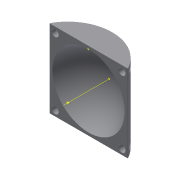
# Autodesk Inventor part: Custom Mirror Design
Saved by Autodesk Inventor 2015 (Build 190159000, 159)
## iProperties
Created: 2014-09-05
Part Number: Custom Mirror Design
Material: Generic
Document SubType Name: Modeling
Designer: I Rabey
Density: 1 g/cm^3
Appearance: Default
Author: I Rabey
Autodesk Inventor part; units mm, degrees
ref_plane "YZ Plane" through (0, 0, 0) normal (1, 0, 0) x (0, 1, 0)
sketch "Sketch11" plane through (0, 0, 0) normal (0, 0, 1) x (1, 0, 0)
  line L0 (-65, -65) -> (65, -65)
  line L1 (65, -65) -> (65, 65)
  line L2 (65, 65) -> (-65, 65)
  line L3 (-65, 65) -> (-65, -65)
  line L4 (-65, -65) -> (65, 65) construction
  line L5 (65, -65) -> (-65, 65) construction
  point P0 (0, 0)
  dimension "d36" = 130
  dimension "d37" = 130
  constraints: 12 end point, 2 midpoint, 2 parallel, 1 horizontal, 1 perpendicular
  measures "d36" distance of L2.end L1.end
  measures "d37" distance of L1.end L0.end
extrude "Extrusion5" add sketch "Sketch11" against normal blind 150
sketch "Sketch12" plane through (0, 0, 0) normal (0, 0, 1) x (1, 0, 0)
  arc A0 (0, 75) -> (0, -75) centre (0, 0) ccw
  line L0 (0, 0) -> (0, 75) construction
  line L1 (0, 0) -> (75, 0) construction
  line L2 (0, 0) -> (0, -75) construction
  line L3 (0, 75) -> (0, -75)
  dimension "d40" = 75
  dimension "d41" = 90
  dimension "d42" = 180
  constraints: 8 end point, 2 point on circle, 1 centre point, 1 coincident, 1 horizontal, 1 perpendicular
  measures "d40" radius of A0
  measures "d41" angle of L1 L0
  measures "d42" angle of L2 L0
revolve "Revolution5" cut sketch "Sketch12" angle 180 about axis through (0, 0, 0) along (0, -1, 0)
ref_plane "Work Plane2" through (0, 65, -37.4166) normal (0, 0, 1) x (1, 0, 0)
sketch "Sketch13" plane through (0, 65, -37.4166) normal (0, 0, 1) x (1, 0, 0)
  line L0 (-65, -130) -> (65, -130)
  line L1 (65, -130) -> (65, 0)
  line L2 (65, 0) -> (-65, 0)
  line L3 (-65, 0) -> (-65, -130)
  line L4 (-65, -130) -> (65, 0) construction
  line L5 (65, -130) -> (-65, 0) construction
  point P0 (0, -65)
  dimension "d45" = 130
  dimension "d46" = 130
  constraints: 12 end point, 2 midpoint, 2 parallel, 1 horizontal, 1 perpendicular
  measures "d45" distance of L2.end L1.end
  measures "d46" distance of L1.end L0.end
extrude "Extrusion6" cut sketch "Sketch13" along normal blind 50
sketch "Sketch14" plane through (0, 65, -37.4166) normal (0, 0, 1) x (1, 0, 0)
  line L0 (-65, -130) -> (65, -130)
  line L1 (65, -130) -> (65, 0)
  line L2 (65, 0) -> (-65, 0)
  line L3 (-65, 0) -> (-65, -130)
  line L4 (-65, -130) -> (65, 0) construction
  line L5 (65, -130) -> (-65, 0) construction
  line L6 (-70, -135) -> (70, -135)
  line L7 (70, -135) -> (70, 5)
  line L8 (70, 5) -> (-70, 5)
  line L9 (-70, 5) -> (-70, -135)
  line L10 (-70, -135) -> (70, 5) construction
  line L11 (70, -135) -> (-70, 5) construction
  point P0 (0, -65)
  dimension "d49" = 130
  dimension "d50" = 130
  dimension "d51" = 140
  dimension "d52" = 140
  constraints: 24 end point, 4 midpoint, 4 parallel, 2 horizontal, 2 perpendicular
  measures "d49" distance of L2.end L1.end
  measures "d50" distance of L1.end L0.end
  measures "d51" distance of L8.end L7.end
  measures "d52" distance of L7.end L6.end
extrude "Extrusion7" add sketch "Sketch14" against normal blind 75
sketch "Sketch17" plane through (0, 0, 0) normal (1, 0, 0) x (0, 1, 0)
  arc A0 (-80, 0) -> (80, 0) centre (0, 0) ccw
  line L0 (0, 0) -> (80, 0) construction
  line L1 (0, 0) -> (80, 0) construction
  line L2 (0, 0) -> (-80, 0) construction
  dimension "d57" = 80
  dimension "d58" = 0
  dimension "d59" = 180
  constraints: 6 end point, 2 point on circle, 1 centre point, 1 coincident, 1 collinear, 1 horizontal
  measures "d57" radius of A0
  measures "d58" distance between parallel lines of L0 L1
  measures "d59" angle of L2 L0
sketch "Sketch18" plane through (-65, 65, -150) normal (0, 1, 0) x (1, 0, 0)
  line L0 (0, -37.5834) -> (130, -37.5834)
  line L1 (130, -37.5834) -> (130, 0)
  line L2 (130, 0) -> (0, 0)
  line L3 (0, 0) -> (0, -37.5834)
  point P0 (65, -150)
  constraints: 8 end point, 2 parallel, 1 horizontal, 1 perpendicular
extrude "Extrusion9" cut sketch "Sketch18" against normal blind 140
ref_plane "Work Plane3" through (0, 0, 0) normal (0, 1, 0) x (-1, 0, 0)
sketch "Sketch22" plane through (0, 0, 0) normal (0, 1, 0) x (-1, 0, 0)
  arc A0 (-65, -37.4166) -> (65, -37.4166) centre (0, 0) ccw projected
  line L0 (0, -75) -> (0, 0)
  circle A1 centre (0, 0) radius 80
  circle A2 centre (0, 0) radius 150
  dimension "d74" = 160
  dimension "d75" = 300
  constraints: 2 centre point, 2 coincident, 2 end point, 1 point on circle, 1 vertical
  measures "d74" diameter of A1
  measures "d75" diameter of A2
extrude "Extrusion10" cut sketch "Sketch22" against normal blind 100 and the other way blind 100
sketch "Sketch24" plane through (0, 65, -37.4166) normal (0, 0, 1) x (1, 0, 0)
  circle A0 centre (-60.1041, -4.8959) radius 2
  point P0 (0, -65)
  dimension "d80" = 4
  dimension "d81" = 85
  dimension "d85" = 60.1041
  constraints: 1 centre point
  measures "d80" diameter of A0
  measures "d81" distance of point (0, -65) A0.centre
  measures "d85" horizontal distance of point (0, -65) A0.centre
sketch "Sketch25" plane through (0, 65, -37.4166) normal (0, 0, 1) x (1, 0, 0)
  circle A0 centre (60.1041, -4.8959) radius 2
  point P0 (0, -65)
  dimension "d82" = 4
  dimension "d83" = 85
  dimension "d84" = 60.1041
  constraints: 1 centre point
  measures "d82" diameter of A0
  measures "d83" distance of point (0, -65) A0.centre
  measures "d84" horizontal distance of point (0, -65) A0.centre
sketch "Sketch26" plane through (0, 65, -37.4166) normal (0, 0, 1) x (1, 0, 0)
  circle A0 centre (-60.1041, -125.1041) radius 2
  point P0 (0, -65)
  dimension "d86" = 4
  dimension "d87" = 85
  dimension "d88" = 60.1041
  constraints: 1 centre point
  measures "d86" diameter of A0
  measures "d87" distance of point (0, -65) A0.centre
  measures "d88" horizontal distance of point (0, -65) A0.centre
sketch "Sketch27" plane through (0, 65, -37.4166) normal (0, 0, 1) x (1, 0, 0)
  circle A0 centre (60.1041, -125.1041) radius 2
  point P0 (0, -65)
  dimension "d89" = 4
  dimension "d90" = 85
  dimension "d91" = 60.1041
  constraints: 1 centre point
  measures "d89" diameter of A0
  measures "d90" distance of A0.centre point (0, -65)
  measures "d91" horizontal distance of point (0, -65) A0.centre
hole "Hole1" at (-60.1041, 60.1041, -37.4166) direction (0, 0, -1) diameter 12.5 end through all
hole "Hole2" at (60.1041, 60.1041, -37.4166) direction (0, 0, -1) diameter 12.5 end through all
hole "Hole3" at (60.1041, -60.1041, -37.4166) direction (0, 0, -1) diameter 12.5 end through all
hole "Hole4" at (-60.1041, -60.1041, -37.4166) direction (0, 0, -1) diameter 12.5 end through all
equation "\"d37\" = d36"
equation "\"d46\" = d45"
body "Solid4"
